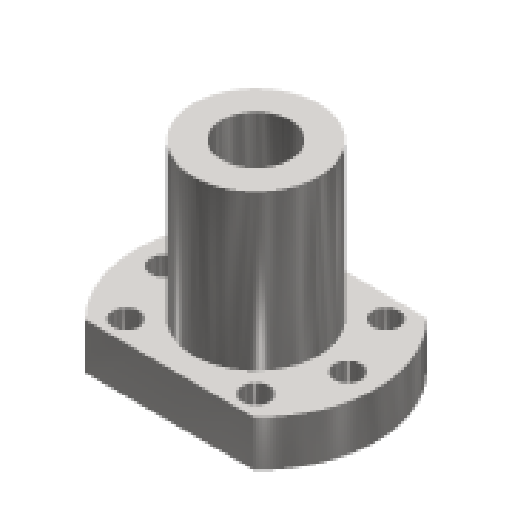
# Autodesk Inventor part: Z Axis Ball Screw Bearing
Saved by Autodesk Inventor 2023.2 (Build 272271000, 271)
## iProperties
Created: 2023-02-17
Part Number: Z Axis Ball Screw Bearing
Material: Stainless Steel
Document SubType Name: Modeling
Designer: remop
Density: 8 g/cm^3
Appearance: Semi-Polished
Author: remop
Autodesk Inventor part; units mm, degrees
ref_plane "YZ Plane" through (0, 0, 0) normal (1, 0, 0) x (0, 1, 0)
ref_plane "XZ Plane" through (0, 0, 0) normal (0, 1, 0) x (-1, 0, 0)
ref_plane "XY Plane" through (0, 0, 0) normal (0, 0, 1) x (1, 0, 0)
sketch "Sketch1" plane through (0, 0, 0) normal (0, 1, 0) x (-1, 0, 0)
  circle A0 centre (0, 0) radius 21
  line L0 (14.6969, -15) -> (-14.6969, -15)
  line L1 (14.6969, 15) -> (-14.6969, 15)
  circle A1 centre (16, 0) radius 2.4
  circle A2 centre (11.3137, 11.3137) radius 2.4
  circle A3 centre (0, 16) radius 2.4
  circle A4 centre (-11.3137, 11.3137) radius 2.4
  circle A5 centre (-16, 0) radius 2.4
  circle A6 centre (-11.3137, -11.3137) radius 2.4
  circle A7 centre (0, -16) radius 2.4
  circle A8 centre (11.3137, -11.3137) radius 2.4
  circle A9 centre (0, 0) radius 6
  point P0 (0, -15)
  point P1 (-2.1817, -15)
  point P2 (2.1817, -15)
  point P3 (2.1817, 15)
  point P4 (-2.1817, 15)
  dimension "d0" = 42
  dimension "d1" = 30
  dimension "d2" = 16
  dimension "d3" = 4.8
  dimension "d6" = 360
  dimension "d10" = 12
  constraints: 10 centre point, 4 end point, 4 point on circle, 2 coincident, 2 parallel, 1 horizontal, 1 horizontal alignment, 1 midpoint, 17 other
  measures "d0" diameter of A0
  measures "d1" distance from line of point (0, -15) L1
  measures "d2" distance of point (0, 0) A1.centre
  measures "d3" diameter of A1
  measures "d10" diameter of A9
extrude "Extrusion1" add sketch "Sketch1" along normal blind 8 contours A0 L0 A7 L1 A3 | A3 L1 | L0 A7 picked at (-0.181, 14.5541) picked at (0.633, -14.8441)
sketch "Sketch2" plane through (0, 8, 0) normal (0, 1, 0) x (1, 0, 0)
  line L0 (14.6969, 15) -> (-14.6969, 15) projected
  arc A0 (-14.6969, 15) -> (-14.6969, -15) centre (0, 0) ccw projected
  line L1 (-14.6969, -15) -> (14.6969, -15) projected
  arc A1 (14.6969, -15) -> (14.6969, 15) centre (0, 0) ccw projected
  circle A2 centre (0, 0) radius 6 projected
  circle A3 centre (-11.3137, 11.3137) radius 2.4 projected
  circle A4 centre (11.3137, 11.3137) radius 2.4 projected
  circle A5 centre (16, 0) radius 2.4 projected
  circle A6 centre (11.3137, -11.3137) radius 2.4 projected
  circle A7 centre (-11.3137, -11.3137) radius 2.4 projected
  circle A8 centre (-16, 0) radius 2.4 projected
  circle A9 centre (0, 0) radius 11
  dimension "d11" = 22
  constraints: 1 centre point, 1 coincident
  measures "d11" diameter of A9
extrude "Extrusion2" add sketch "Sketch2" along normal blind 27 contours A9
body "Solid1"
